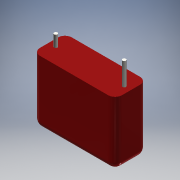
# Autodesk Inventor part: MKP4 0,1µF 630VDC (450377)
Saved by Autodesk Inventor 2017 (Build 210142000, 142)
## iProperties
Part Number: MKP4 0,1µF 630VDC (450377)
Material: Generisch
Document SubType Name: Modeling
Designer: David Merges
Density: 1 g/cm^3
Appearance: Rot
Author: David Merges
Autodesk Inventor part; units mm, degrees
ref_plane "YZ Plane" through (0, 0, 0) normal (1, 0, 0) x (0, 1, 0)
ref_plane "XZ Plane" through (0, 0, 0) normal (0, 1, 0) x (-1, 0, 0)
ref_plane "XY Plane" through (0, 0, 0) normal (0, 0, 1) x (1, 0, 0)
sketch "Skizze1" plane through (0, 0, 0) normal (0, 0, 1) x (1, 0, 0)
  line L0 (-9, 3.5) -> (9, 3.5)
  line L1 (9, 3.5) -> (9, -3.5)
  line L2 (9, -3.5) -> (-9, -3.5)
  line L3 (-9, -3.5) -> (-9, 3.5)
  line L4 (9, -3.5) -> (-9, 3.5) construction
  point P0 (0, 0)
  point P1 (0, 0)
  dimension "d0" = 18
  dimension "d1" = 7
  constraints: 10 end point, 2 parallel, 1 coincident, 1 horizontal, 1 midpoint, 1 perpendicular
  measures "d0" distance of L0.start L0.end
  measures "d1" distance of L2.end L0.start
extrude "Extrusion1" add sketch "Skizze1" along normal blind 14
sketch "Skizze2" plane through (0, 0, 14) normal (0, 0, 1) x (1, 0, 0)
  circle A0 centre (-7.5, 0) radius 0.375
  circle A1 centre (7.5, 0) radius 0.375
  line L0 (7.5, 0) -> (-7.5, 0) construction
  point P0 (0, 0)
  point P1 (0, 0)
  dimension "d4" = 15
  dimension "d5" = 0.75
  constraints: 2 centre point, 2 end point, 1 coincident, 1 equal radius, 1 horizontal, 1 midpoint
  measures "d4" distance of L0.start L0.end
  measures "d5" diameter of A0
extrude "Extrusion2" add sketch "Skizze2" along normal blind 5
fillet "Rundung1" radius 1.5 4 edges at (9, -3.5, 7) (-9, -3.5, 7) (9, 3.5, 7) (-9, 3.5, 7)
fillet "Rundung2" radius 1.5 8 edges at (-8.5607, -3.0607, 0) (-9, 0, 0) (-8.5607, 3.0607, 0) (0, 3.5, 0) (8.5607, 3.0607, 0) (9, 0, 0) (8.5607, -3.0607, 0) (0, -3.5, 0)
sketch "Skizze3" plane through (-7.5, 0, 19) normal (0, 0, 1) x (1, 0, 0)
  circle A0 centre (0, 0) radius 0.375 projected
  circle A1 centre (15, 0) radius 0.375 projected
  point P0 (7.5, 0)
extrude "Extrusion3" cut sketch "Skizze3" against normal blind 2.5 contours A0
